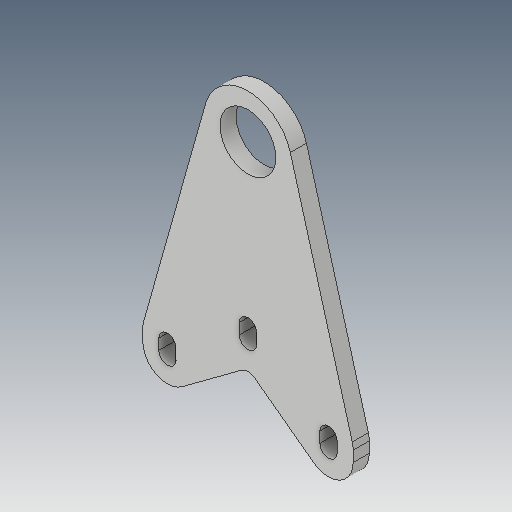
# Autodesk Inventor part: POT2BASE
Saved by Autodesk Inventor 2019.4 (Build 234330000, 330)
## iProperties
Created: 2019-06-16
Part Number: POT2BASE
Material: Generic
Document SubType Name: Modeling
Designer: AzLIer
Density: 1 g/cm^3
Appearance: Default
Mass: 3.66853 g
Surface Area: 31.5994 cm^2
Volume: 3.66853 cm^3
Author: AzLIer
Autodesk Inventor part; units mm, degrees
ref_plane "YZ Plane" through (0, 0, 0) normal (1, 0, 0) x (0, 1, 0)
ref_plane "XZ Plane" through (0, 0, 0) normal (0, 1, 0) x (-1, 0, 0)
ref_plane "XY Plane" through (0, 0, 0) normal (0, 0, 1) x (1, 0, 0)
sketch "スケッチ1" plane through (0, 0, 0) normal (0, 0, 1) x (1, 0, 0)
  line L0 (0, 0) -> (0, -2) construction
  line L1 (-1.6, 0) -> (-1.6, -2)
  line L2 (1.6, -2) -> (1.6, 0)
  arc A0 (1.6, 0) -> (-1.6, 0) centre (0, 0) ccw
  arc A1 (-1.6, -2) -> (1.6, -2) centre (0, -2) ccw
  line L3 (-30, -50) -> (30, -50)
  line L4 (30, -50) -> (30, 50)
  line L5 (30, 50) -> (-30, 50)
  line L6 (-30, 50) -> (-30, -50)
  line L7 (-30, -50) -> (30, 50) construction
  line L8 (30, -50) -> (-30, 50) construction
  line L9 (15, -10) -> (-15, -10) construction
  line L10 (15, -10) -> (15, -12) construction
  line L11 (13.4, -10) -> (13.4, -12)
  line L12 (16.6, -12) -> (16.6, -10)
  arc A2 (16.6, -10) -> (13.4, -10) centre (15, -10) ccw
  arc A3 (13.4, -12) -> (16.6, -12) centre (15, -12) ccw
  line L13 (-15, -10) -> (-15, -12) construction
  line L14 (-16.6, -10) -> (-16.6, -12)
  line L15 (-13.4, -12) -> (-13.4, -10)
  arc A4 (-13.4, -10) -> (-16.6, -10) centre (-15, -10) ccw
  arc A5 (-16.6, -12) -> (-13.4, -12) centre (-15, -12) ccw
  point P0 (0, -1)
  point P1 (15, -11)
  point P2 (-15, -11)
  point P3 (0, -10)
  dimension "d0" = 3.2
  dimension "d1" = 60
  dimension "d2" = 100
  dimension "d5" = 30
  dimension "d6" = 10
  dimension "d7" = 2
  constraints: 38 end point, 12 point on circle, 12 tangent, 8 parallel, 7 midpoint, 6 centre point, 2 equal radius, 2 horizontal, 2 perpendicular, 1 vertical, 1 vertical alignment
  measures "d0" diameter of A1
  measures "d1" distance of L5.end L4.end
  measures "d2" distance of L4.end L3.end
  measures "d5" distance of L9.start L9.end
  measures "d6" distance from line of L0.start L9
  measures "d7" distance of L0.start L0.end
extrude "押し出し1" add sketch "スケッチ1" along normal blind 3
sketch "スケッチ2" plane through (0, 0, 3) normal (0, 0, 1) x (1, 0, 0)
  arc A0 (2.0211, 340.4082) -> (8.8067, 38.5424) centre (32.0275, 190.0735) ccw projected
  circle A1 centre (0, 29.945) radius 10 construction
  circle A2 centre (0, 29.945) radius 5.2
  arc A3 (-13.4, -10) -> (-16.6, -10) centre (-15, -10) ccw projected
  line L0 (-13.4, -10) -> (-13.4, -12) projected
  arc A4 (-16.6, -12) -> (-13.4, -12) centre (-15, -12) ccw projected
  line L1 (-16.6, -12) -> (-16.6, -10) projected
  arc A5 (16.6, -10) -> (13.4, -10) centre (15, -10) ccw projected
  line L2 (16.6, -10) -> (16.6, -12) projected
  arc A6 (13.4, -12) -> (16.6, -12) centre (15, -12) ccw projected
  line L3 (13.4, -12) -> (13.4, -10) projected
  arc A7 (1.6, 0) -> (-1.6, 0) centre (0, 0) ccw projected
  line L4 (1.6, 0) -> (1.6, -2) projected
  arc A8 (-1.6, -2) -> (1.6, -2) centre (0, -2) ccw projected
  line L5 (-1.6, -2) -> (-1.6, 0) projected
  line L6 (-30, -50) -> (30, -50) projected
  line L7 (30, -50) -> (30, 50) projected
  line L8 (30, 50) -> (-30, 50) projected
  line L9 (-30, 50) -> (-30, -50) projected
  arc A9 (19.6, -10) -> (19.4275, -8.752) centre (15, -10) ccw
  line L10 (19.6, -10) -> (19.6, -12)
  arc A10 (12.2593, -15.6944) -> (19.6, -12) centre (15, -12) ccw
  line L11 (10.4, -12) -> (10.4, -10)
  line L12 (4.6, -2) -> (4.6, 0)
  arc A11 (4.6, 0) -> (-4.6, 0) centre (0, 0) ccw
  line L13 (-4.6, 0) -> (-4.6, -2)
  arc A12 (-4.6, -2) -> (4.6, -2) centre (0, -2) ccw
  arc A13 (-19.4275, -8.752) -> (-19.6, -10) centre (-15, -10) ccw
  line L14 (-10.4, -10) -> (-10.4, -12)
  arc A14 (-19.6, -12) -> (-12.2593, -15.6944) centre (-15, -12) ccw
  line L15 (-19.6, -12) -> (-19.6, -10)
  arc A15 (7.8924, 32.1697) -> (-7.8924, 32.1697) centre (0, 29.945) ccw
  line L16 (19.4275, -8.752) -> (7.8924, 32.1697)
  line L17 (-19.4275, -8.752) -> (-7.8924, 32.1697)
  line L18 (0, -6.6) -> (12.2593, -15.6944)
  line L19 (0, -6.6) -> (-12.2593, -15.6944)
  dimension "d8" = 20
  dimension "d9" = 10.4
  dimension "d10" = 3
  dimension "d11" = 3
  dimension "d12" = 3
  dimension "d13" = 3
  constraints: 20 end point, 15 point on circle, 9 centre point, 7 tangent, 1 coincident, 1 vertical alignment, 3 other
  measures "d8" diameter of A1
  measures "d9" diameter of A2
  measures "d10" radial gap between concentric circles of A5 A9
  measures "d11" radial gap between concentric circles of A8 A12
  measures "d12" radial gap between concentric circles of A3 A13
  measures "d13" radial gap between concentric circles of A2 A15
extrude "押し出し2" cut sketch "スケッチ2" against normal blind 3 contours A12 L13 A11 L12 | L10 A10 L18 L19 A14 L15 A13 L17 A15 L16 A9 keep common part
fillet "フィレット1" radius 2 1 edges at (0, -6.6, 1.5)
